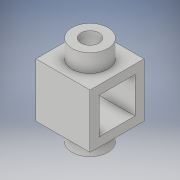
# Autodesk Inventor part: Osa_rameno _1
Saved by Autodesk Inventor 2018.2 (Build 222227000, 227)
## iProperties
Created: 2018-03-10
Part Number: Osa_rameno _1
Material: Všeobecné
Document SubType Name: Modeling
Designer: Lukáš
Density: 1 g/cm^3
Appearance: Výchozí
Author: Lukáš
Autodesk Inventor part; units mm, degrees
ref_plane "YZ Plane" through (0, 0, 0) normal (1, 0, 0) x (0, 1, 0)
ref_plane "XZ Plane" through (0, 0, 0) normal (0, 1, 0) x (-1, 0, 0)
ref_plane "XY Plane" through (0, 0, 0) normal (0, 0, 1) x (1, 0, 0)
sketch "Náčrt1" plane through (0, 0, 0) normal (0, 0, 1) x (1, 0, 0)
  line L0 (4.5, 0) -> (4.5, -4.5)
  line L1 (4.5, -4.5) -> (-4.5, -4.5)
  line L2 (-4.5, -4.5) -> (-4.5, 4.5)
  line L3 (-4.5, 4.5) -> (4.5, 4.5)
  line L4 (4.5, 4.5) -> (4.5, -4.5)
  circle A0 centre (0, 0) radius 3
  circle A1 centre (0, 0) radius 1.5
  dimension "d1" = 4.5
  dimension "d2" = 9
  dimension "d3" = 9
  dimension "d4" = 9
  dimension "d5" = 6
  dimension "d6" = 3
  constraints: 10 end point, 2 centre point, 2 coincident, 2 perpendicular, 1 collinear, 1 point on line
  measures "d1" distance of L0.start L0.end
  measures "d2" distance of L0.end L1.end
  measures "d3" distance of L1.end L2.end
  measures "d4" distance of L2.end L3.end
  measures "d5" diameter of A0
  measures "d6" diameter of A1
extrude "Vysunutí1" add sketch "Náčrt1" along normal blind 9 contours L0 L1 L2 L3 L4 | A0 | A1
sketch "Náčrt2" plane through (0, 0, 9) normal (0, 0, 1) x (1, 0, 0)
  circle A0 centre (0, 0) radius 3
  circle A1 centre (0, 0) radius 1.5
  dimension "d9" = 6
  dimension "d10" = 3
  constraints: 2 centre point, 2 coincident
  measures "d9" diameter of A0
  measures "d10" diameter of A1
extrude "Vysunutí2" add sketch "Náčrt2" along normal blind 3
sketch "Náčrt3" plane through (0, 0, 0) normal (0, 0, -1) x (-1, 0, 0)
  circle A0 centre (0, 0) radius 3
  circle A1 centre (0, 0) radius 1.5
  dimension "d13" = 6
  dimension "d14" = 3
  constraints: 2 centre point, 2 coincident
  measures "d13" diameter of A0
  measures "d14" diameter of A1
extrude "Vysunutí3" add sketch "Náčrt3" along normal blind 3
sketch "Náčrt4" plane through (-4.5, -4.5, 0) normal (-1, 0, 0) x (0, 0, 1)
  line L0 (0, 9) -> (0, 0) projected
  line L1 (0, 0) -> (9, 0) projected
  line L2 (1.5, 0) -> (1.5, 1.5)
  line L3 (1.5, 1.5) -> (1.5, 7.5)
  line L4 (1.5, 7.5) -> (7.5, 7.5)
  line L5 (7.5, 7.5) -> (7.5, 1.5)
  line L6 (7.5, 1.5) -> (1.5, 1.5)
  point P0 (0, 4.5)
  dimension "d18" = 1.5
  dimension "d19" = 6
  dimension "d20" = 6
  dimension "d21" = 6
  constraints: 10 end point, 2 perpendicular, 2 point on line
  measures "d18" distance of L2.start L2.end
  measures "d19" distance of L2.end L3.end
  measures "d20" distance of L3.end L4.end
  measures "d21" distance of L4.end L5.end
extrude "Vysunutí4" cut sketch "Náčrt4" against normal blind 9
